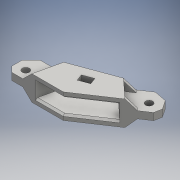
# Autodesk Inventor part: Support_GP2.Ar
Saved by Autodesk Inventor 2016 (Build 200138000, 138)
## iProperties
Created: 2016-09-30
Part Number: Support_GP2.Ar
Material: Générique
Document SubType Name: Modeling
Designer: LogOut
Density: 1 g/cm^3
Appearance: Par défaut
Author: LogOut
Autodesk Inventor part; units mm, degrees
ref_plane "YZ Plane" through (0, 0, 0) normal (1, 0, 0) x (0, 1, 0)
ref_plane "XZ Plane" through (0, 0, 0) normal (0, 1, 0) x (-1, 0, 0)
ref_plane "XY Plane" through (0, 0, 0) normal (0, 0, 1) x (1, 0, 0)
sketch "Esquisse1" plane through (0, 0, 0) normal (0, 0, 1) x (1, 0, 0)
  line L0 (-170, -60) -> (-110, -100)
  line L1 (-156, 0) -> (-156, -52.507427)
  line L2 (-156, 0) -> (-156, 51.347524)
  line L3 (-90, 100) -> (-170, 60)
  line L4 (-170, 60) -> (-170, -60)
  line L5 (156, 0) -> (156, 51.347524)
  line L6 (110, -100) -> (170, -60)
  line L7 (170, 60) -> (90, 100)
  line L8 (-78.695048, 90) -> (-54, 90)
  line L9 (-54, 100) -> (-69, 100)
  line L10 (-156, 51.347524) -> (-78.695048, 90)
  line L11 (-54, -90) -> (-54, 100)
  line L12 (-54, 100) -> (-81.055728, 100)
  line L13 (-81.055728, 100) -> (-166, 57.527864)
  line L14 (-166, 57.527864) -> (-166, 0)
  line L15 (-166, 0) -> (-166, -52.507427)
  line L16 (-54, 80) -> (-76.334369, 80)
  line L17 (-76.334369, 80) -> (-156, 40.167184)
  line L18 (-146, 45.167184) -> (-146, 0)
  line L19 (-146, 0) -> (-146, -52.507427)
  line L20 (-156, 51.347524) -> (-160.472136, 60.291796)
  line L21 (-156, 51.347524) -> (-151.527864, 42.403252)
  line L22 (99.761141, -90) -> (156, -52.507427)
  line L23 (54, -90) -> (99.761141, -90)
  line L24 (150.452998, -44.186924) -> (96.733385, -80)
  line L25 (96.733385, -80) -> (54, -80)
  line L26 (161.547002, -60.82793) -> (102.788897, -100)
  line L27 (102.788897, -100) -> (54, -100)
  line L28 (54, -80) -> (54, -100)
  line L29 (150.452998, -44.186924) -> (161.547002, -60.82793)
  point P0 (0, 0)
  dimension "d0" = 14
  dimension "d2" = 10
  dimension "d6" = 56
  dimension "d8" = 14
  dimension "d10" = 14
  dimension "d11" = 14
  dimension "d12" = 10
  dimension "d13" = 10
  dimension "d15" = 10
  dimension "d16" = 10
  constraints: 60 end point, 7 point on line, 4 vertical, 2 horizontal, 2 parallel, 2 perpendicular, 5 other
  measures "d0" distance from line of L4 L1.start
  measures "d2" distance between parallel lines of L8 L9
  measures "d6" horizontal distance of L0.end L11.start
  measures "d8" distance from line of L7 L5.end
  measures "d10" distance from line of L0 L1.end
  measures "d11" distance from line of L3 L10.start
  measures "d12" distance between parallel lines of L10 L13
  measures "d13" distance between parallel lines of L10 L17
  measures "d15" distance between parallel lines of L22 L24
  measures "d16" distance between parallel lines of L22 L26
extrude "Extrusion1" add sketch "Esquisse1" along normal blind 28 contours L23 L28 L25 L24 L29 L22 | L22 L29 L26 L27 L28 L23
move faces "Déplacer1" translate (-12, 0, 0) faces at (54, -86.666667, 9.333333)
move faces "Déplacer2" translate (9.984604, 6.656402, 0) faces at (157.849001, -55.280928, 9.333333)
sketch "Esquisse2" plane through (0, 0, 28) normal (0, 0, 1) x (1, 0, 0)
  line L0 (42, -80) -> (42, -100)
  line L1 (42, -90) -> (54, -90)
  line L2 (171.531605, -54.171528) -> (160.437602, -37.530522)
  line L3 (165.984604, -45.851025) -> (156, -52.507427)
  point P0 (0, 0)
  dimension "d25" = 12
  dimension "d26" = 12
  constraints: 4 end point, 2 midpoint, 1 horizontal, 1 perpendicular
  measures "d25" distance of L1.start L1.end
  measures "d26" distance from line of L2 L3.end
hole "Perçage1" at (54, -90, 28) at (156, -52.507427, 28) direction (0, 0, -1) diameter 8 end through all
move faces "Déplacer3" translate (0, 8, 0) faces at (78.488923, -80, 9.333333)
move faces "Déplacer4" translate (-3.328201, 4.992302, 0) faces at (143.202863, -49.020348, 18.666667)
move faces "Déplacer5" translate (1.1094, -1.664101, 0) faces at (148.617369, -69.447685, 18.666667)
sketch "Esquisse3" plane through (0, 0, 28) normal (0, 0, 1) x (1, 0, 0)
  circle A0 centre (54, -90) radius 4
  circle A1 centre (156, -52.507427) radius 4
  line L0 (54, -90) -> (156, -52.507427)
  line L1 (50.549946, -80.613993) -> (152.549946, -43.121421)
  line L2 (50.549946, -80.613993) -> (69.290015, -84.379784)
  line L3 (152.549946, -43.121421) -> (146.144621, -56.130011)
  point P0 (0, 0)
  dimension "d43" = 10
  constraints: 8 end point, 2 point on line, 1 parallel
  measures "d43" distance between parallel lines of L0 L1
extrude "Extrusion2" add sketch "Esquisse3" against normal blind 28 contours L2 L1 L3 L0
ref_plane "Plan de construction1" through (75.36467, -75.754403, 28) normal (-0.3450054, 0.9386007, 0) x (0.9386007, 0.3450054, 0)
sketch "Esquisse4" plane through (75.36467, -75.754403, 28) normal (-0.3450054, 0.9386007, 0) x (0.9386007, 0.3450054, 0)
  line L0 (0, 0) -> (0, 28)
  line L1 (0, 0) -> (56.83331, 0)
  line L2 (56.83331, 28) -> (56.83331, 0)
  line L3 (0, 28) -> (56.83331, 28)
  line L4 (6, 6) -> (54, 6)
  line L5 (54, 6) -> (54, 22)
  line L6 (54, 22) -> (6, 22)
  line L7 (6, 22) -> (6, 6)
  point P0 (-44.601651, 28)
  dimension "d47" = 48
  dimension "d48" = 6
  dimension "d49" = 2.83331
  dimension "d50" = 16
  dimension "d51" = 6
  constraints: 8 end point, 2 parallel, 1 horizontal, 1 perpendicular
  measures "d47" distance of L4.start L4.end
  measures "d48" distance between parallel lines of L0 L7
  measures "d49" distance between parallel lines of L2 L5
  measures "d50" distance between parallel lines of L6 L4
  measures "d51" distance between parallel lines of L1 L4
extrude "Extrusion3" cut sketch "Esquisse4" against normal through all contours L7 L6 L5 L4
sketch "Esquisse5" plane through (42, -100, 0) normal (0, -1, 0) x (1, 0, 0)
  line L0 (38.996274, 22) -> (84.049107, 22)
  line L1 (38.996274, 6) -> (38.996274, 22)
  line L2 (84.049107, 6) -> (38.996274, 6)
  line L3 (84.049107, 22) -> (84.049107, 6)
  point P0 (-42, 0)
extrude "Extrusion4" cut sketch "Esquisse5" against normal up to surface surface through (103.522691, -65.40424, 14) normal (-0.3450054, 0.9386007, 0)
sketch "Esquisse6" plane through (172.641006, -55.835629, 0) normal (0.5547002, -0.8320503, 0) x (0.8320503, 0.5547002, 0)
  line L0 (-86.153726, 22) -> (-39.481523, 22)
  line L1 (-86.153726, 6) -> (-86.153726, 22)
  line L2 (-39.481523, 6) -> (-86.153726, 6)
  line L3 (-39.481523, 22) -> (-39.481523, 6)
  point P0 (-112.673966, 0)
extrude "Extrusion5" cut sketch "Esquisse6" against normal up to surface surface through (103.522691, -65.40424, 14) normal (-0.3450054, 0.9386007, 0)
sketch "Esquisse7" plane through (75.36467, -75.754403, 28) normal (0.3450054, -0.9386007, 0) x (0.9386007, 0.3450054, 0)
  line L0 (11.5, -14) -> (48.5, -14)
  line L1 (6, -22) -> (6, -6) projected
  line L2 (54, -22) -> (6, -22) projected
  point P0 (-44.601651, -28)
  dimension "d58" = 37
  dimension "d59" = 5.5
  dimension "d60" = 8
  constraints: 2 end point, 1 horizontal
  measures "d58" distance of L0.start L0.end
  measures "d59" distance from line of L1 L0.start
  measures "d60" distance between parallel lines of L2 L0
hole "Perçage2" at (86.158578, -71.78684, 14) at (120.886804, -59.021639, 14) direction (-0.3450054, 0.9386007, 0) diameter 4 end through all
sketch "Esquisse9" plane through (42, -100, 0) normal (0, -1, 0) x (1, 0, 0)
  line L0 (32.996274, 22) -> (38.996274, 22)
  line L1 (38.996274, 22) -> (38.996274, 6)
  line L2 (38.996274, 6) -> (32.996274, 6)
  line L3 (32.996274, 6) -> (32.996274, 22)
  line L4 (38.996274, 6) -> (38.996274, 22)
  line L5 (38.996274, 22) -> (64.394449, 22)
  line L6 (64.394449, 6) -> (38.996274, 6)
  point P0 (-42, 0)
  dimension "d72" = 6
  constraints: 8 end point, 3 collinear, 2 parallel, 1 horizontal, 1 perpendicular
  measures "d72" distance between parallel lines of L1 L3
extrude "Extrusion7" cut sketch "Esquisse9" against normal up to surface surface through (103.522691, -65.40424, 14) normal (-0.3450054, 0.9386007, 0)
chamfer "Chanfrein1" distance 6.392 distance2 24.11 1 edges at (74.9963, -75.8898, 14) measured on face at (75.4656, -75.7173, 14)
sketch "Esquisse11" plane through (172.641006, -55.835629, 0) normal (0.5547002, -0.8320503, 0) x (0.8320503, 0.5547002, 0)
  line L0 (-33.481523, 22) -> (-39.481523, 22)
  line L1 (-39.481523, 22) -> (-39.481523, 6)
  line L2 (-39.481523, 6) -> (-33.481523, 6)
  line L3 (-33.481523, 6) -> (-33.481523, 22)
  line L4 (-79.618453, 22) -> (-39.481523, 22)
  line L5 (-39.481523, 6) -> (-79.618453, 6)
  line L6 (-39.481523, 22) -> (-39.481523, 6)
  point P0 (-112.673966, 0)
  dimension "d78" = 6
  constraints: 8 end point, 3 collinear, 2 parallel, 1 horizontal, 1 perpendicular
  measures "d78" distance between parallel lines of L6 L3
extrude "Extrusion8" cut sketch "Esquisse11" against normal up to surface surface through (103.522691, -65.40424, 14) normal (-0.3450054, 0.9386007, 0)
chamfer "Chanfrein2" distance 6.171 distance2 23.331 1 edges at (131.8409, -54.9952, 14) measured on face at (131.3716, -55.1677, 14)
sketch "Esquisse12" plane through (0, 0, 28) normal (0, 0, 1) x (1, 0, 0)
  line L0 (80.99581, -73.684541) -> (74.996274, -99.999816)
  line L1 (74.996274, -99.999816) -> (80.99581, -73.684541)
  line L2 (126.048823, -57.124214) -> (144.782638, -74.407751)
  line L3 (144.782638, -74.407751) -> (126.048823, -57.124214)
  line L4 (77.578387, -70.679034) -> (70.893593, -100)
  line L5 (126.96393, -52.526181) -> (148.207156, -72.124862)
  line L6 (73.984649, -72) -> (42, -72)
  line L7 (42, -72) -> (42, -100)
  line L8 (42, -100) -> (106.394449, -100)
  line L9 (106.394449, -100) -> (172.641006, -55.835629)
  line L10 (172.641006, -55.835629) -> (157.1094, -32.53822)
  line L11 (157.1094, -32.53822) -> (127.328432, -52.392199)
  line L12 (73.984649, -72) -> (127.328432, -52.392199)
  circle A0 centre (54, -90) radius 4
  circle A1 centre (156, -52.507427) radius 4
  point P0 (0, 0)
  dimension "d84" = 4
  dimension "d85" = 4
  constraints: 4 end point, 4 point on line, 2 parallel
  measures "d84" distance between parallel lines of L0 L4
  measures "d85" distance between parallel lines of L2 L5
extrude "Extrusion9" cut sketch "Esquisse12" against normal blind 10 contours L4 L8 L7 L6 L12 | L12 L11 L10 L9 L5
ref_plane "Plan de construction2" through (74.996274, -100, 14) normal (0, 0, 1) x (1, 0, 0)
mirror "Symétrie1" about plane through (74.996274, -100, 14) normal (0, 0, 1) of "Extrusion9"
chamfer "Chanfrein3" distance 10 angle 45 4 edges at (137.5855, -62.3255, 18) (137.5855, -62.3255, 10) (74.236, -85.3395, 18) (74.236, -85.3395, 10)
sketch "Esquisse13" plane through (0, 0, 28) normal (0, 0, 1) x (1, 0, 0)
  line L0 (73.984649, -72) -> (67.020626, -72)
  line L1 (77.578387, -70.679034) -> (73.984649, -72)
  line L2 (60.636995, -100) -> (70.893593, -100)
  line L3 (127.328432, -52.392199) -> (135.59363, -46.882067)
  line L4 (148.207156, -72.124862) -> (156.768258, -66.417461)
  line L5 (66.108679, -76) -> (74.696513, -76)
  line L6 (74.696513, -76) -> (76.517914, -75.3305)
  line L7 (61.548943, -96) -> (71.80554, -96)
  line L8 (130.057475, -55.380239) -> (138.618577, -49.672837)
  line L9 (145.182209, -69.334091) -> (153.743311, -63.62669)
  line L10 (126.96393, -52.526181) -> (127.328432, -52.392199)
  line L11 (148.207156, -72.124862) -> (126.96393, -52.526181)
  line L12 (148.207156, -72.124862) -> (156.768258, -66.417461)
  line L13 (156.768258, -66.417461) -> (135.59363, -46.882067)
  line L14 (127.328432, -52.392199) -> (135.59363, -46.882067)
  line L15 (73.984649, -72) -> (67.020626, -72)
  line L16 (67.020626, -72) -> (60.636995, -100)
  line L17 (60.636995, -100) -> (70.893593, -100)
  line L18 (77.578387, -70.679034) -> (70.893593, -100)
  line L19 (77.578387, -70.679034) -> (73.984649, -72)
  point P0 (0, 0)
  dimension "d92" = 4
  dimension "d93" = 4
  dimension "d94" = 4
  dimension "d95" = 4
  constraints: 10 end point, 8 point on line, 3 parallel
  measures "d92" distance between parallel lines of L0 L5
  measures "d93" distance between parallel lines of L2 L7
  measures "d94" distance between parallel lines of L3 L8
  measures "d95" distance between parallel lines of L4 L9
extrude "Extrusion10" cut sketch "Esquisse13" against normal blind 10 contours L5 L6 L18 L7 L16 | L13 L9 L11 L8
mirror "Symétrie2" about plane through (74.996274, -100, 14) normal (0, 0, 1) of "Extrusion10"
chamfer "Chanfrein4" distance 2 angle 45 10 edges at (74.9963, -99.9999, 22) (90.6954, -100, 22) (144.7827, -74.4078, 22) (125.5886, -87.2039, 22) (74.9963, -99.9999, 6) (90.6954, -100, 6) (144.7827, -74.4078, 6) (125.5886, -87.2039, 6) (84.7786, -68.0324, 16) (119.5068, -55.2672, 16)
chamfer "Chanfrein5" distance 6 angle 45 2 edges at (42, -100, 14) (172.641, -55.8356, 14)
chamfer "Chanfrein6" distance 10 angle 45 2 edges at (42, -72, 14) (157.1094, -32.5382, 14)
sketch "Esquisse14" plane through (105.788897, -98, 22) normal (0, 0, -1) x (-1, 0, 0)
  line L0 (30.336691, 0) -> (0, 0)
  line L1 (30.336691, 0) -> (24.793087, 24.315459)
  line L2 (24.793087, 24.315459) -> (-20.259925, 40.875786)
  line L3 (-20.259925, 40.875786) -> (-37.481344, 24.987563)
  line L4 (0, 0) -> (-37.481344, 24.987563)
  line L5 (5.828242, 24.893953) -> (-5.434966, 29.034018)
  line L6 (-5.434966, 29.034018) -> (-8.195009, 21.525213)
  line L7 (-8.195009, 21.525213) -> (3.068199, 17.385147)
  line L8 (3.068199, 17.385147) -> (5.828242, 24.893953)
  point P0 (105.788897, 98)
  dimension "d107" = 6
  dimension "d108" = 8
  dimension "d109" = 12
  dimension "d110" = 18
  dimension "d111" = 18.00019
  constraints: 8 end point, 3 parallel, 1 perpendicular
  measures "d107" distance between parallel lines of L2 L5
  measures "d108" distance between parallel lines of L5 L7
  measures "d109" distance between parallel lines of L8 L6
  measures "d110" distance from line of L1.end L8
  measures "d111" distance from line of L2.end L6
extrude "Extrusion11" cut sketch "Esquisse14" against normal blind 10 contours L8 L7 L6 L5
chamfer "Chanfrein7" distance 8 distance2 6 1 edges at (108.3523, -78.5448, 22) measured on face at (108.5248, -79.0141, 22)
